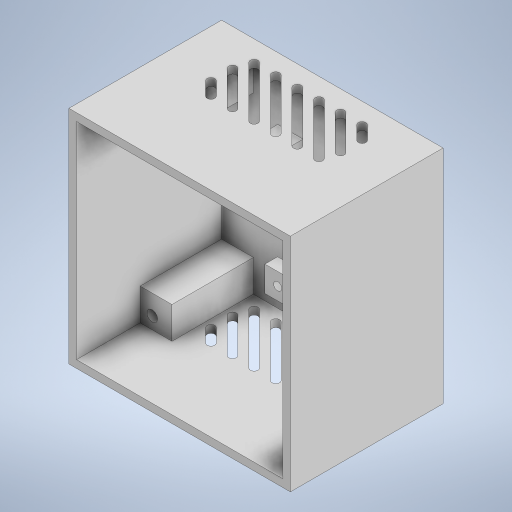
# Autodesk Inventor part: Temp_controller_box
Saved by Autodesk Inventor 2024 (Build 280153000, 153)
## iProperties
Created: 2026-04-14
Part Number: Temp_controller_box
Material: Generic
Document SubType Name: Modeling
Designer: Péter
Density: 1 g/cm^3
Appearance: Default
Author: Péter
Autodesk Inventor part; units mm, degrees
ref_plane "YZ Plane" through (0, 0, 0) normal (1, 0, 0) x (0, 1, 0)
sketch "Sketch1" plane through (0, 0, 0) normal (0, 0, 1) x (1, 0, 0)
  line L0 (-43.5, 43.5) -> (43.5, 43.5)
  line L1 (43.5, 43.5) -> (43.5, -43.5)
  line L2 (43.5, -43.5) -> (-43.5, -43.5)
  line L3 (-43.5, -43.5) -> (-43.5, 43.5)
  line L4 (-43.5, 43.5) -> (43.5, -43.5) construction
  line L5 (43.5, 43.5) -> (-43.5, -43.5) construction
  point P0 (0, 0)
  dimension "d0" = 87
  dimension "d1" = 87
  constraints: 12 end point, 2 midpoint, 2 parallel, 1 horizontal, 1 perpendicular
  measures "d0" distance of L1.end L2.end
  measures "d1" distance of L0.end L1.end
extrude "Extrusion1" add sketch "Sketch1" along normal blind 60
shell "Shell1" thickness 3 removed faces 1 at (-14.5, 14.5, 60)
sketch "Sketch2" plane through (-40.5, -40.5, 3) normal (0, 0, 1) x (1, 0, 0)
  line L0 (22, 62.5) -> (32, 62.5)
  line L1 (32, 62.5) -> (32, 52.5)
  line L2 (32, 52.5) -> (22, 52.5)
  line L3 (22, 52.5) -> (22, 62.5)
  line L4 (22, 62.5) -> (32, 52.5) construction
  line L5 (32, 62.5) -> (22, 52.5) construction
  line L6 (52, 62.5) -> (62, 62.5)
  line L7 (62, 62.5) -> (62, 52.5)
  line L8 (62, 52.5) -> (52, 52.5)
  line L9 (52, 52.5) -> (52, 62.5)
  line L10 (52, 62.5) -> (62, 52.5) construction
  line L11 (62, 62.5) -> (52, 52.5) construction
  line L12 (22, 17.5) -> (32, 17.5)
  line L13 (32, 17.5) -> (32, 7.5)
  line L14 (32, 7.5) -> (22, 7.5)
  line L15 (22, 7.5) -> (22, 17.5)
  line L16 (22, 17.5) -> (32, 7.5) construction
  line L17 (32, 17.5) -> (22, 7.5) construction
  line L18 (62, 17.5) -> (52, 17.5)
  line L19 (52, 17.5) -> (52, 7.5)
  line L20 (52, 7.5) -> (62, 7.5)
  line L21 (62, 7.5) -> (62, 17.5)
  line L22 (62, 17.5) -> (52, 7.5) construction
  line L23 (52, 17.5) -> (62, 7.5) construction
  line L24 (27, 57.5) -> (57, 57.5) construction
  line L25 (57, 12.5) -> (27, 12.5) construction
  line L26 (27, 57.5) -> (27, 12.5) construction
  line L27 (57, 12.5) -> (57, 57.5) construction
  line L28 (0, 0) -> (0, 81) projected
  line L29 (0, 81) -> (81, 81) projected
  line L30 (-3, 84) -> (-3, -3) projected
  line L31 (81, 0) -> (0, 0) projected
  point P0 (40.5, 40.5)
  dimension "d5" = 10
  dimension "d6" = 10
  dimension "d7" = 10
  dimension "d8" = 10
  dimension "d9" = 10
  dimension "d10" = 10
  dimension "d11" = 10
  dimension "d12" = 10
  dimension "d13" = 30
  dimension "d14" = 45
  dimension "d15" = 30
  dimension "d42" = 7.5
  constraints: 56 end point, 11 parallel, 8 midpoint, 5 perpendicular, 4 horizontal
  measures "d5" distance of L1.end L2.end
  measures "d6" distance of L0.end L1.end
  measures "d7" distance of L7.end L8.end
  measures "d8" distance of L6.end L7.end
  measures "d9" distance of L13.end L14.end
  measures "d10" distance of L12.end L13.end
  measures "d11" distance of L20.end L19.end
  measures "d12" distance of L19.end L18.end
  measures "d13" distance of L25.start L25.end
  measures "d14" distance of L25.start L24.end
  measures "d15" distance between parallel lines of L30 L26
  measures "d42" distance between parallel lines of L31 L14
extrude "Extrusion2" add sketch "Sketch2" along normal blind 5
sketch "Sketch3" plane through (-40.5, -40.5, 8) normal (0, 0, 1) x (1, 0, 0)
  line L0 (57, 57.5) -> (27, 57.5) construction
  line L1 (27, 57.5) -> (27, 12.5) construction
  line L2 (27, 12.5) -> (57, 12.5) construction
  line L3 (57, 12.5) -> (57, 57.5) construction
  line L4 (0, 81) -> (81, 81) projected
  line L5 (81, 81) -> (81, 0) projected
  line L6 (22, 17.5) -> (22, 7.5) projected
  line L7 (22, 7.5) -> (32, 7.5) projected
  line L8 (62, 7.5) -> (62, 17.5) projected
  point P0 (40.5, 40.5)
  dimension "d19" = 5
  dimension "d20" = 5
  dimension "d21" = 5
  dimension "d22" = 45
  constraints: 8 end point, 4 parallel, 1 horizontal, 1 perpendicular
  measures "d19" distance between parallel lines of L6 L1
  measures "d20" distance between parallel lines of L7 L2
  measures "d21" distance between parallel lines of L8 L3
  measures "d22" distance of L2.end L0.start
hole "Hole1" at (-13.5, 17, 8) at (-13.5, -28, 8) at (16.5, -28, 8) at (16.5, 17, 8) direction (0, 0, -1) diameter 3.2 end through all
sketch "Sketch4" plane through (0, 0, 0) normal (0, 0, -1) x (-1, 0, 0)
  circle A0 centre (-16.5, 17) radius 1.6 projected
  line L0 (-14.8834, 19.8) -> (-13.2668, 17)
  line L1 (-13.2668, 17) -> (-14.8834, 14.2)
  line L2 (-14.8834, 14.2) -> (-18.1166, 14.2)
  line L3 (-18.1166, 14.2) -> (-19.7332, 17)
  line L4 (-19.7332, 17) -> (-18.1166, 19.8)
  line L5 (-18.1166, 19.8) -> (-14.8834, 19.8)
  circle A1 centre (13.5, 17) radius 1.6 projected
  line L6 (15.1166, 19.8) -> (16.7332, 17)
  line L7 (16.7332, 17) -> (15.1166, 14.2)
  line L8 (15.1166, 14.2) -> (11.8834, 14.2)
  line L9 (11.8834, 14.2) -> (10.2668, 17)
  line L10 (10.2668, 17) -> (11.8834, 19.8)
  line L11 (11.8834, 19.8) -> (15.1166, 19.8)
  circle A2 centre (13.5, -28) radius 1.6 projected
  line L12 (15.1166, -25.2) -> (16.7332, -28)
  line L13 (16.7332, -28) -> (15.1166, -30.8)
  line L14 (15.1166, -30.8) -> (11.8834, -30.8)
  line L15 (11.8834, -30.8) -> (10.2668, -28)
  line L16 (10.2668, -28) -> (11.8834, -25.2)
  line L17 (11.8834, -25.2) -> (15.1166, -25.2)
  circle A3 centre (-16.5, -28) radius 1.6 projected
  line L18 (-14.8834, -25.2) -> (-13.2668, -28)
  line L19 (-13.2668, -28) -> (-14.8834, -30.8)
  line L20 (-14.8834, -30.8) -> (-18.1166, -30.8)
  line L21 (-18.1166, -30.8) -> (-19.7332, -28)
  line L22 (-19.7332, -28) -> (-18.1166, -25.2)
  line L23 (-18.1166, -25.2) -> (-14.8834, -25.2)
  line L24 (-43.5, 43.5) -> (43.5, 43.5) projected
  point P0 (0, 0)
  dimension "d30" = 5.6
  dimension "d31" = 5.6
  dimension "d32" = 5.6
  constraints: 48 end point, 4 coincident, 3 parallel, 1 collinear, 1 point on line, 52 other
  measures "d30" distance between parallel lines of L23 L20
  measures "d31" distance between parallel lines of L17 L14
  measures "d32" distance between parallel lines of L5 L2
extrude "Extrusion3" cut sketch "Sketch4" against normal blind 5
ref_plane "Work Plane1" through (0, 0, 35) normal (0, 0, 1) x (1, 0, 0)
sketch "Sketch6" plane through (0, 0, 35) normal (0, 0, 1) x (1, 0, 0)
  line L0 (40.5, -40.5) -> (40.5, 40.5) projected
  line L1 (40.5, -40.5) -> (28, -40.5)
  line L2 (28, -40.5) -> (28, -28)
  line L3 (28, -28) -> (40.5, -28)
  line L4 (40.5, -28) -> (40.5, -40.5)
  line L5 (-40.5, -40.5) -> (-40.5, 40.5) projected
  line L6 (-40.5, -40.5) -> (-28, -40.5)
  line L7 (-28, -40.5) -> (-28, -28)
  line L8 (-28, -28) -> (-40.5, -28)
  line L9 (-40.5, -28) -> (-40.5, -40.5)
  line L10 (40.5, 40.5) -> (28, 40.5)
  line L11 (28, 40.5) -> (28, 28)
  line L12 (28, 28) -> (40.5, 28)
  line L13 (40.5, 28) -> (40.5, 40.5)
  line L14 (-40.5, 40.5) -> (-28, 40.5)
  line L15 (-28, 40.5) -> (-28, 28)
  line L16 (-28, 28) -> (-40.5, 28)
  line L17 (-40.5, 28) -> (-40.5, 40.5)
  point P0 (0, 0)
  point P1 (40.5, 28)
  point P2 (40.5, -28)
  dimension "d44" = 12.5
  dimension "d45" = 12.5
  dimension "d46" = 12.5
  dimension "d47" = 12.5
  dimension "d48" = 12.5
  dimension "d49" = 12.5
  dimension "d50" = 12.5
  dimension "d51" = 12.5
  constraints: 32 end point, 8 parallel, 4 horizontal, 4 perpendicular
  measures "d44" distance of L2.end L3.end
  measures "d45" distance of L1.end L2.end
  measures "d46" distance of L8.end L7.end
  measures "d47" distance of L7.end L6.end
  measures "d48" distance of L12.end L11.end
  measures "d49" distance of L11.end L10.end
  measures "d50" distance of L15.end L16.end
  measures "d51" distance of L14.end L15.end
extrude "Extrusion5" add sketch "Sketch6" against normal up to surface (32 mm away)
sketch "Sketch7" plane through (0, 0, 35) normal (0, 0, 1) x (1, 0, 0)
  line L0 (35.75, 35.75) -> (-35.75, 35.75) construction
  line L1 (-35.75, 35.75) -> (-35.75, -35.75) construction
  line L2 (-35.75, -35.75) -> (35.75, -35.75) construction
  line L3 (35.75, -35.75) -> (35.75, 35.75) construction
  line L4 (-40.5, -40.5) -> (-40.5, 40.5) projected
  line L5 (40.5, -40.5) -> (-40.5, -40.5) projected
  line L6 (40.5, 40.5) -> (40.5, -40.5) projected
  line L7 (-40.5, 40.5) -> (40.5, 40.5) projected
  point P0 (0, 0)
  dimension "d65" = 71.5
  dimension "d66" = 71.5
  dimension "d67" = 35.75
  dimension "d68" = 35.75
  constraints: 8 end point, 6 parallel, 1 vertical
  measures "d65" distance of L1.end L2.end
  measures "d66" distance of L2.end L0.start
  measures "d67" distance from line of point (0, 0) L1
  measures "d68" distance from line of point (0, 0) L2
hole "Hole2" at (35.75, -35.75, 35) at (-35.75, -35.75, 35) at (-35.75, 35.75, 35) at (35.75, 35.75, 35) direction (0, 0, -1) diameter 4.2 end through all
sketch "Sketch8" plane through (-43.5, -43.5, 0) normal (0, -1, 0) x (1, 0, 0)
  line L0 (18.5, 28) -> (68.5, 28) construction
  line L1 (68.5, 28) -> (68.5, 8) construction
  line L2 (68.5, 8) -> (18.5, 8) construction
  line L3 (18.5, 8) -> (18.5, 28) construction
  line L4 (0, 0) -> (87, 0) projected
  line L5 (0, 0) -> (0, 60) projected
  line L6 (18.5, 22.6967) -> (23.8033, 28) construction
  line L7 (17.4393, 23.7574) -> (22.7426, 29.0607)
  line L8 (24.864, 26.9393) -> (19.5607, 21.636)
  arc A0 (17.4393, 23.7574) -> (19.5607, 21.636) centre (18.5, 22.6967) ccw
  arc A1 (24.864, 26.9393) -> (22.7426, 29.0607) centre (23.8033, 28) ccw
  line L9 (18.5, 14.2114) -> (32.2886, 28) construction
  line L10 (17.4393, 15.2721) -> (31.2279, 29.0607)
  line L11 (33.3492, 26.9393) -> (19.5607, 13.1508)
  arc A2 (17.4393, 15.2721) -> (19.5607, 13.1508) centre (18.5, 14.2114) ccw
  arc A3 (33.3492, 26.9393) -> (31.2279, 29.0607) centre (32.2886, 28) ccw
  line L12 (20.7739, 8) -> (40.7739, 28) construction
  line L13 (19.7132, 9.0607) -> (39.7132, 29.0607)
  line L14 (41.8345, 26.9393) -> (21.8345, 6.9393)
  arc A4 (19.7132, 9.0607) -> (21.8345, 6.9393) centre (20.7739, 8) ccw
  arc A5 (41.8345, 26.9393) -> (39.7132, 29.0607) centre (40.7739, 28) ccw
  line L15 (29.2591, 8) -> (49.2591, 28) construction
  line L16 (28.1985, 9.0607) -> (48.1985, 29.0607)
  line L17 (50.3198, 26.9393) -> (30.3198, 6.9393)
  arc A6 (28.1985, 9.0607) -> (30.3198, 6.9393) centre (29.2591, 8) ccw
  arc A7 (50.3198, 26.9393) -> (48.1985, 29.0607) centre (49.2591, 28) ccw
  line L18 (37.7444, 8) -> (57.7444, 28) construction
  line L19 (36.6838, 9.0607) -> (56.6838, 29.0607)
  line L20 (58.8051, 26.9393) -> (38.8051, 6.9393)
  arc A8 (36.6838, 9.0607) -> (38.8051, 6.9393) centre (37.7444, 8) ccw
  arc A9 (58.8051, 26.9393) -> (56.6838, 29.0607) centre (57.7444, 28) ccw
  line L21 (46.2297, 8) -> (66.2297, 28) construction
  line L22 (45.169, 9.0607) -> (65.169, 29.0607)
  line L23 (67.2904, 26.9393) -> (47.2904, 6.9393)
  arc A10 (45.169, 9.0607) -> (47.2904, 6.9393) centre (46.2297, 8) ccw
  arc A11 (67.2904, 26.9393) -> (65.169, 29.0607) centre (66.2297, 28) ccw
  line L24 (54.715, 8) -> (68.5, 21.785) construction
  line L25 (53.6543, 9.0607) -> (67.4393, 22.8457)
  line L26 (69.5607, 20.7244) -> (55.7756, 6.9393)
  arc A12 (53.6543, 9.0607) -> (55.7756, 6.9393) centre (54.715, 8) ccw
  arc A13 (69.5607, 20.7244) -> (67.4393, 22.8457) centre (68.5, 21.785) ccw
  line L27 (63.2003, 8) -> (68.5, 13.2997) construction
  line L28 (62.1396, 9.0607) -> (67.4393, 14.3604)
  line L29 (69.5607, 12.2391) -> (64.2609, 6.9393)
  arc A14 (62.1396, 9.0607) -> (64.2609, 6.9393) centre (63.2003, 8) ccw
  arc A15 (69.5607, 12.2391) -> (67.4393, 14.3604) centre (68.5, 13.2997) ccw
  point P0 (43.5, 0)
  point P1 (21.1517, 25.3483)
  point P2 (43.5, 0)
  dimension "d69" = 8
  dimension "d70" = 20
  dimension "d71" = 50
  dimension "d73" = 3
  dimension "d74" = 45
  dimension "d75" = 3
  dimension "d76" = 3
  dimension "d77" = 3
  dimension "d78" = 3
  dimension "d79" = 3
  dimension "d80" = 3
  dimension "d81" = 6
  dimension "d82" = 6
  dimension "d83" = 6
  dimension "d84" = 6
  dimension "d85" = 6
  dimension "d86" = 6
  dimension "d87" = 3
  dimension "d88" = 6
  dimension "d89" = 7.5
  dimension "d92" = 25
  constraints: 72 end point, 32 point on circle, 32 tangent, 16 centre point, 16 point on line, 10 parallel, 2 midpoint, 1 horizontal, 1 perpendicular
  measures "d69" distance between parallel lines of L4 L2
  measures "d70" distance of L0.end L1.end
  measures "d71" distance of L0.start L0.end
  measures "d73" distance between parallel lines of L7 L8
  measures "d74" angle of L2 L6
  measures "d75" distance between parallel lines of L10 L11
  measures "d76" distance between parallel lines of L13 L14
  measures "d77" distance between parallel lines of L16 L17
  measures "d78" distance between parallel lines of L19 L20
  measures "d79" distance between parallel lines of L22 L23
  measures "d80" distance between parallel lines of L25 L26
  measures "d81" distance between parallel lines of L9 L6
  measures "d82" distance between parallel lines of L12 L9
  measures "d83" distance between parallel lines of L15 L12
  measures "d84" distance between parallel lines of L15 L18
  measures "d85" distance between parallel lines of L21 L18
  measures "d86" distance between parallel lines of L24 L21
  measures "d87" distance between parallel lines of L28 L29
  measures "d88" distance between parallel lines of L24 L27
  measures "d89" distance of L6.start L6.end
  measures "d92" distance from line of point (43.5, 0) L3
extrude "Extrusion6" cut sketch "Sketch8" against normal up to surface (3 mm away)
ref_plane "Work Plane2" through (-43.5, 0, 0) normal (0, 1, 0) x (1, 0, 0)
mirror "Mirror1" about plane through (-43.5, 0, 0) normal (0, 1, 0) of "Extrusion6"
body "Solid1"
